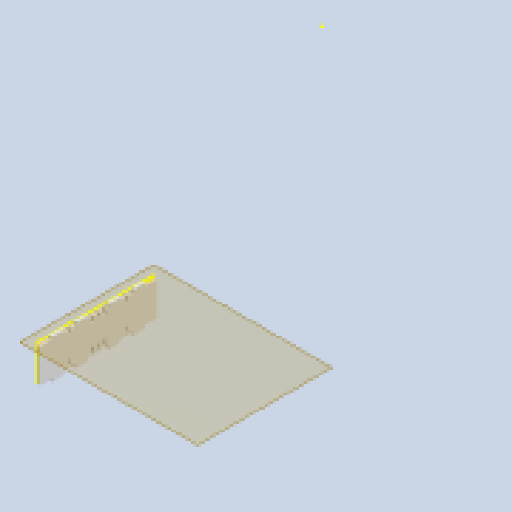
# Autodesk Inventor part: стенка
Saved by Autodesk Inventor 2024.2 (Build 282272000, 272)
## iProperties
Created: 2025-12-09
Part Number: стенка
Material: Типовые
Document SubType Name: Modeling
Designer: katya_notebook
Mass: 65.1748 g
Surface Area: 247.334 cm^2
Volume: 65.1748 cm^3
Density: 1 g/cm^3
Appearance: По умолчанию
Author: katya_notebook
Autodesk Inventor part; units mm, degrees
ref_plane "YZ Plane" through (0, 0, 0) normal (1, 0, 0) x (0, 1, 0)
ref_plane "XZ Plane" through (0, 0, 0) normal (0, 1, 0) x (-1, 0, 0)
ref_plane "XY Plane" through (0, 0, 0) normal (0, 0, 1) x (1, 0, 0)
ref_plane "РабПлоскость1" through (-475.2675, -216.9886, 379.0883) normal (0, 1, 0) x (-1, 0, 0)
sketch "Эскиз1" plane through (-475.2675, -216.9886, 379.0883) normal (0, 1, 0) x (-1, 0, 0)
  line L0 (135, 97.5) -> (129, 97.5)
  line L1 (129, 97.5) -> (129, -97.5)
  line L2 (129, -97.5) -> (135, -97.5)
  line L3 (135, -97.5) -> (135, 97.5)
  line L4 (135, -97.5) -> (135, 97.5) projected
  line L5 (135, 97.5) -> (62.5237, 97.5) projected
  line L6 (62.5237, -97.5) -> (135, -97.5) projected
  point P0 (-475.2675, -379.0883)
  dimension "d0" = 0
  dimension "d1" = 6
  dimension "d2" = 0
  dimension "d3" = 0
  constraints: 8 end point, 2 parallel, 1 horizontal, 1 perpendicular
  measures "d0" distance between parallel lines of L4 L3
  measures "d1" distance of L0.start L0.end
  measures "d2" distance between parallel lines of L6 L2
  measures "d3" distance between parallel lines of L0 L5
ref_plane "РабПлоскость2" through (-610.2675, -276.6936, 277.5883) normal (0, 1, 0) x (0, 0, 1)
extrude "Выдавливание1" add sketch "Эскиз1" against normal up to surface (59.705 mm away)
sketch "Эскиз2" plane through (-610.2675, -216.9886, 281.5883) normal (-1, 0, 0) x (0, 0, 1)
  line L0 (0, -4) -> (20, -4) projected
  line L1 (195, 0) -> (195, -59.705) projected
  line L2 (0, 0) -> (195, 0) projected
  line L3 (0, 0) -> (0, -59.705) projected
  point P0 (-281.5883, 216.9886)
  point P1 (195, -59.705)
  constraints: 1 other
sketch "Эскиз3" plane through (-610.2675, -276.6936, 281.5883) normal (-1, 0, 0) x (0, 0, 1)
  line L0 (195, 0) -> (0, 0) projected
  line L1 (175, 0) -> (155, 0)
  line L2 (155, 0) -> (155, -5)
  line L3 (155, -5) -> (175, -5)
  line L4 (175, -5) -> (175, 0)
  line L5 (195, 59.705) -> (195, 0) projected
  line L6 (135, 0) -> (115, 0)
  line L7 (115, 0) -> (115, -5)
  line L8 (115, -5) -> (135, -5)
  line L9 (135, -5) -> (135, 0)
  line L10 (20, 0) -> (40, 0)
  line L11 (40, 0) -> (40, -5)
  line L12 (40, -5) -> (20, -5)
  line L13 (20, -5) -> (20, 0)
  line L14 (60, 0) -> (80, 0)
  line L15 (80, 0) -> (80, -5)
  line L16 (80, -5) -> (60, -5)
  line L17 (60, -5) -> (60, 0)
  line L18 (97.5, 27.8525) -> (226.4185, 27.8525)
  line L19 (195, 55.705) -> (0, 55.705)
  line L20 (175, 55.705) -> (155, 55.705)
  line L21 (155, 55.705) -> (155, 60.705)
  line L22 (155, 60.705) -> (175, 60.705)
  line L23 (175, 60.705) -> (175, 55.705)
  line L24 (135, 55.705) -> (115, 55.705)
  line L25 (115, 55.705) -> (115, 60.705)
  line L26 (115, 60.705) -> (135, 60.705)
  line L27 (135, 60.705) -> (135, 55.705)
  line L28 (20, 55.705) -> (40, 55.705)
  line L29 (40, 55.705) -> (40, 60.705)
  line L30 (40, 60.705) -> (20, 60.705)
  line L31 (20, 60.705) -> (20, 55.705)
  line L32 (60, 55.705) -> (80, 55.705)
  line L33 (80, 55.705) -> (80, 60.705)
  line L34 (80, 60.705) -> (60, 60.705)
  line L35 (60, 60.705) -> (60, 55.705)
  point P0 (-281.5883, 276.6936)
  point P1 (40, 55.705)
  point P2 (80, 55.705)
  point P3 (40, 0)
  point P4 (80, 0)
  point P5 (115, 55.705)
  point P6 (155, 55.705)
  point P7 (115, 0)
  point P8 (155, 0)
  dimension "d8" = 5
  dimension "d9" = 20
  dimension "d10" = 20
  dimension "d11" = 20
  dimension "d12" = 20
  dimension "d13" = 5
  dimension "d14" = 20
  dimension "d15" = 20
  dimension "d16" = 20
  dimension "d17" = 20
  dimension "d43" = 5
  constraints: 68 end point, 17 symmetric about line, 8 parallel, 8 point on line, 5 horizontal, 4 perpendicular
  measures "d8" distance of L3.end L1.start
  measures "d9" distance of L2.end L3.end
  measures "d10" distance of L0.start L1.start
  measures "d11" distance of L7.end L8.end
  measures "d12" distance of L1.end L6.start
  measures "d13" distance of L10.end L11.end
  measures "d14" distance of L11.end L12.end
  measures "d15" distance of L10.start L0.end
  measures "d16" distance of L15.end L16.end
  measures "d17" distance of L14.start L10.end
  measures "d43" distance of L16.end L14.start
extrude "Выдавливание3" add sketch "Эскиз3" against normal blind 6
sketch "Эскиз4" plane through (-610.2675, -276.6936, 281.5883) normal (-1, 0, 0) x (0, 0, 1)
  point P0 (-281.5883, 276.6936)
sketch "Эскиз5" plane through (-610.2675, -276.6936, 281.5883) normal (-1, 0, 0) x (0, 0, 1)
  point P0 (-281.5883, 276.6936)
sketch "Эскиз6" plane through (-610.2675, -276.6936, 281.5883) normal (-1, 0, 0) x (0, 0, 1)
  line L0 (111.125, 1.5) -> (104.625, 1.5)
  line L1 (104.625, 1.5) -> (104.625, 4.5)
  line L2 (104.625, 4.5) -> (111.125, 4.5)
  line L3 (111.125, 4.5) -> (111.125, 1.5)
  line L4 (115, 0) -> (115, -5) projected
  line L5 (100.75, 1.5) -> (94.25, 1.5)
  line L6 (94.25, 1.5) -> (94.25, 4.5)
  line L7 (94.25, 4.5) -> (100.75, 4.5)
  line L8 (100.75, 4.5) -> (100.75, 1.5)
  line L9 (90.375, 1.5) -> (83.875, 1.5)
  line L10 (83.875, 1.5) -> (83.875, 4.5)
  line L11 (83.875, 4.5) -> (90.375, 4.5)
  line L12 (90.375, 4.5) -> (90.375, 1.5)
  line L13 (111.125, 3) -> (104.625, 3)
  line L14 (115, 0) -> (80, 0) projected
  line L15 (106.125, 6) -> (109.625, 6)
  line L16 (109.625, 6) -> (109.625, 0)
  line L17 (109.625, 0) -> (106.125, 0)
  line L18 (106.125, 0) -> (106.125, 6)
  line L19 (106.125, 6) -> (109.625, 0) construction
  line L20 (109.625, 6) -> (106.125, 0) construction
  line L21 (100.75, 3) -> (94.25, 3)
  line L22 (97.5, 1.5) -> (97.5, 4.5)
  line L23 (90.375, 3) -> (83.875, 3)
  line L24 (87.125, 1.5) -> (87.125, 4.5)
  line L25 (95.75, 6) -> (99.25, 6)
  line L26 (99.25, 6) -> (99.25, 0)
  line L27 (99.25, 0) -> (95.75, 0)
  line L28 (95.75, 0) -> (95.75, 6)
  line L29 (95.75, 6) -> (99.25, 0) construction
  line L30 (99.25, 6) -> (95.75, 0) construction
  line L31 (85.375, 6) -> (88.875, 6)
  line L32 (88.875, 6) -> (88.875, 0)
  line L33 (88.875, 0) -> (85.375, 0)
  line L34 (85.375, 0) -> (85.375, 6)
  line L35 (85.375, 6) -> (88.875, 0) construction
  line L36 (88.875, 6) -> (85.375, 0) construction
  line L37 (148.25, 1.5) -> (141.75, 1.5)
  line L38 (141.75, 1.5) -> (141.75, 4.5)
  line L39 (141.75, 4.5) -> (148.25, 4.5)
  line L40 (148.25, 4.5) -> (148.25, 1.5)
  line L41 (148.25, 3) -> (141.75, 3)
  line L42 (143.25, 12) -> (146.75, 12)
  line L43 (146.75, 12) -> (146.75, -6)
  line L44 (146.75, -6) -> (143.25, -6)
  line L45 (143.25, -6) -> (143.25, 12)
  line L46 (143.25, 12) -> (146.75, -6) construction
  line L47 (146.75, 12) -> (143.25, -6) construction
  line L48 (155, 0) -> (155, -5) projected
  line L49 (53.25, 1.5) -> (46.75, 1.5)
  line L50 (46.75, 1.5) -> (46.75, 4.5)
  line L51 (46.75, 4.5) -> (53.25, 4.5)
  line L52 (53.25, 4.5) -> (53.25, 1.5)
  line L53 (53.25, 3) -> (46.75, 3)
  line L54 (48.25, 12) -> (51.75, 12)
  line L55 (51.75, 12) -> (51.75, -6)
  line L56 (51.75, -6) -> (48.25, -6)
  line L57 (48.25, -6) -> (48.25, 12)
  line L58 (48.25, 12) -> (51.75, -6) construction
  line L59 (51.75, 12) -> (48.25, -6) construction
  line L60 (60, 0) -> (60, -5) projected
  line L61 (195, 59.705) -> (195, 0) projected
  line L62 (195, 29.8525) -> (88.875, 29.8525)
  line L63 (111.125, 58.205) -> (104.625, 58.205)
  line L64 (104.625, 58.205) -> (104.625, 55.205)
  line L65 (104.625, 55.205) -> (111.125, 55.205)
  line L66 (111.125, 55.205) -> (111.125, 58.205)
  line L67 (115, 59.705) -> (115, 64.705)
  line L68 (100.75, 58.205) -> (94.25, 58.205)
  line L69 (94.25, 58.205) -> (94.25, 55.205)
  line L70 (94.25, 55.205) -> (100.75, 55.205)
  line L71 (100.75, 55.205) -> (100.75, 58.205)
  line L72 (90.375, 58.205) -> (83.875, 58.205)
  line L73 (83.875, 58.205) -> (83.875, 55.205)
  line L74 (83.875, 55.205) -> (90.375, 55.205)
  line L75 (90.375, 55.205) -> (90.375, 58.205)
  line L76 (111.125, 56.705) -> (104.625, 56.705)
  line L77 (115, 59.705) -> (80, 59.705)
  line L78 (106.125, 53.705) -> (109.625, 53.705)
  line L79 (109.625, 53.705) -> (109.625, 59.705)
  line L80 (109.625, 59.705) -> (106.125, 59.705)
  line L81 (106.125, 59.705) -> (106.125, 53.705)
  line L82 (106.125, 53.705) -> (109.625, 59.705) construction
  line L83 (109.625, 53.705) -> (106.125, 59.705) construction
  line L84 (100.75, 56.705) -> (94.25, 56.705)
  line L85 (97.5, 58.205) -> (97.5, 55.205)
  line L86 (90.375, 56.705) -> (83.875, 56.705)
  line L87 (87.125, 58.205) -> (87.125, 55.205)
  line L88 (95.75, 53.705) -> (99.25, 53.705)
  line L89 (99.25, 53.705) -> (99.25, 59.705)
  line L90 (99.25, 59.705) -> (95.75, 59.705)
  line L91 (95.75, 59.705) -> (95.75, 53.705)
  line L92 (95.75, 53.705) -> (99.25, 59.705) construction
  line L93 (99.25, 53.705) -> (95.75, 59.705) construction
  line L94 (85.375, 53.705) -> (88.875, 53.705)
  line L95 (88.875, 53.705) -> (88.875, 59.705)
  line L96 (88.875, 59.705) -> (85.375, 59.705)
  line L97 (85.375, 59.705) -> (85.375, 53.705)
  line L98 (85.375, 53.705) -> (88.875, 59.705) construction
  line L99 (88.875, 53.705) -> (85.375, 59.705) construction
  line L100 (146.75, 65.705) -> (143.25, 65.705)
  line L101 (146.75, 47.705) -> (146.75, 65.705)
  line L102 (146.75, 47.705) -> (143.25, 65.705) construction
  line L103 (143.25, 47.705) -> (146.75, 65.705) construction
  line L104 (143.25, 65.705) -> (143.25, 47.705)
  line L105 (141.75, 58.205) -> (141.75, 55.205)
  line L106 (148.25, 58.205) -> (141.75, 58.205)
  line L107 (148.25, 55.205) -> (148.25, 58.205)
  line L108 (141.75, 55.205) -> (148.25, 55.205)
  line L109 (148.25, 56.705) -> (141.75, 56.705)
  line L110 (143.25, 47.705) -> (146.75, 47.705)
  line L111 (155, 59.705) -> (155, 64.705)
  line L112 (51.75, 65.705) -> (48.25, 65.705)
  line L113 (51.75, 47.705) -> (51.75, 65.705)
  line L114 (51.75, 47.705) -> (48.25, 65.705) construction
  line L115 (48.25, 47.705) -> (51.75, 65.705) construction
  line L116 (48.25, 65.705) -> (48.25, 47.705)
  line L117 (46.75, 58.205) -> (46.75, 55.205)
  line L118 (53.25, 58.205) -> (46.75, 58.205)
  line L119 (53.25, 55.205) -> (53.25, 58.205)
  line L120 (46.75, 55.205) -> (53.25, 55.205)
  line L121 (53.25, 56.705) -> (46.75, 56.705)
  line L122 (48.25, 47.705) -> (51.75, 47.705)
  line L123 (60, 59.705) -> (60, 64.705)
  line L124 (109.625, 6) -> (106.125, 6)
  line L125 (106.125, 6) -> (106.125, 12)
  line L126 (106.125, 12) -> (109.625, 12)
  line L127 (109.625, 12) -> (109.625, 6)
  line L128 (99.25, 6) -> (95.75, 6)
  line L129 (95.75, 6) -> (95.75, 12)
  line L130 (95.75, 12) -> (99.25, 12)
  line L131 (99.25, 12) -> (99.25, 6)
  line L132 (88.875, 6) -> (85.375, 6)
  line L133 (85.375, 6) -> (85.375, 12)
  line L134 (85.375, 12) -> (88.875, 12)
  line L135 (88.875, 12) -> (88.875, 6)
  line L136 (109.625, 53.705) -> (106.125, 53.705)
  line L137 (106.125, 53.705) -> (106.125, 47.705)
  line L138 (106.125, 47.705) -> (109.625, 47.705)
  line L139 (109.625, 47.705) -> (109.625, 53.705)
  line L140 (99.25, 53.705) -> (95.75, 53.705)
  line L141 (95.75, 53.705) -> (95.75, 47.705)
  line L142 (95.75, 47.705) -> (99.25, 47.705)
  line L143 (99.25, 47.705) -> (99.25, 53.705)
  line L144 (88.875, 53.705) -> (85.375, 53.705)
  line L145 (85.375, 53.705) -> (85.375, 47.705)
  line L146 (85.375, 47.705) -> (88.875, 47.705)
  line L147 (88.875, 47.705) -> (88.875, 53.705)
  point P0 (-281.5883, 276.6936)
  point P1 (115, -2.5)
  point P2 (107.875, 11.6549)
  point P3 (107.875, 3)
  point P4 (97.5, 3)
  point P5 (87.125, 3)
  point P6 (149.0518, 14.6563)
  point P7 (145, 3)
  point P8 (155, -2.5)
  point P9 (49.2049, 25.9501)
  point P10 (50, 3)
  point P11 (60, -2.5)
  point P12 (48.25, 4.5)
  point P13 (48.25, 1.5)
  point P14 (51.75, 1.5)
  point P15 (51.75, 4.5)
  point P16 (88.875, 4.5)
  point P17 (85.375, 4.5)
  point P18 (85.375, 1.5)
  point P19 (85.375, 0)
  point P20 (88.875, 1.5)
  point P21 (95.75, 1.5)
  point P22 (95.75, 0)
  point P23 (99.25, 1.5)
  point P24 (99.25, 4.5)
  point P25 (95.75, 4.5)
  point P26 (106.125, 1.5)
  point P27 (106.125, 0)
  point P28 (109.625, 1.5)
  point P29 (109.625, 4.5)
  point P30 (106.125, 4.5)
  point P31 (143.25, 1.5)
  point P32 (146.75, 1.5)
  point P33 (146.75, 4.5)
  point P34 (143.25, 4.5)
  point P35 (195, 55.705)
  point P36 (115, 62.205)
  point P37 (107.875, 48.0501)
  point P38 (107.875, 56.705)
  point P39 (97.5, 56.705)
  point P40 (87.125, 56.705)
  point P41 (145, 56.705)
  point P42 (149.0518, 45.0486)
  point P43 (155, 62.205)
  point P44 (50, 56.705)
  point P45 (60, 62.205)
  point P46 (51.75, 55.205)
  point P47 (51.75, 58.205)
  point P48 (48.25, 58.205)
  point P49 (48.25, 55.205)
  point P50 (88.875, 55.205)
  point P51 (88.875, 58.205)
  point P52 (85.375, 55.705)
  point P53 (85.375, 58.205)
  point P54 (85.375, 55.205)
  point P55 (99.25, 55.205)
  point P56 (99.25, 58.205)
  point P57 (95.75, 58.205)
  point P58 (95.75, 55.205)
  point P59 (106.125, 58.205)
  point P60 (106.125, 55.205)
  point P61 (109.625, 55.205)
  point P62 (109.625, 58.205)
  point P63 (143.25, 58.205)
  point P64 (143.25, 55.205)
  point P65 (146.75, 55.205)
  point P66 (146.75, 58.205)
  point P67 (85.375, 59.705)
  point P68 (85.375, 53.705)
  point P69 (95.75, 53.705)
  point P70 (106.125, 53.705)
  point P71 (85.375, 6)
  point P72 (95.75, 6)
  point P73 (106.125, 6)
  dimension "d1" = 6
  dimension "d20" = 6.5
  dimension "d21" = 3
  dimension "d22" = 3.875
  dimension "d23" = 6.5
  dimension "d24" = 3
  dimension "d25" = 3.875
  dimension "d26" = 6.5
  dimension "d27" = 3
  dimension "d28" = 3.875
  dimension "d29" = 3
  dimension "d30" = 3.5
  dimension "d31" = 3.5
  dimension "d32" = 3.5
  dimension "d33" = 6.5
  dimension "d34" = 3
  dimension "d35" = 3.5
  dimension "d36" = 8.25
  dimension "d37" = 6.5
  dimension "d38" = 3
  dimension "d39" = 3.5
  dimension "d40" = 8.25
  dimension "d46" = 6
  dimension "d47" = 6
  constraints: 286 end point, 71 symmetric about line, 33 midpoint, 32 parallel, 18 perpendicular, 17 horizontal, 8 collinear, 8 point on line
  measures "d20" distance of L0.start L0.end
  measures "d21" distance of L0.end L1.end
  measures "d22" horizontal distance of L13.start point (115, -2.5)
  measures "d23" distance of L5.start L5.end
  measures "d24" distance of L5.end L6.end
  measures "d25" distance of L7.end L1.end
  measures "d26" distance of L9.start L9.end
  measures "d27" distance of L9.end L10.end
  measures "d28" distance of L6.end L11.end
  measures "d29" distance from line of L14 point (107.875, 3)
  measures "d30" distance of L16.end L17.end
  measures "d31" distance of L27.end L26.end
  measures "d32" distance of L33.end L32.end
  measures "d33" distance of L37.start L38.start
  measures "d34" distance of L38.start L38.end
  measures "d35" distance of L44.start L44.end
  measures "d36" distance from line of L43 point (155, -2.5)
  measures "d37" distance of L49.start L50.start
  measures "d38" distance of L50.start L50.end
  measures "d39" distance of L56.start L56.end
  measures "d40" distance from line of L55 point (60, -2.5)
  measures "d46" distance of L124.end L125.end
  measures "d47" distance of L136.end L137.end
extrude "Выдавливание4" cut sketch "Эскиз6" against normal blind 6
sketch "Эскиз7" plane through (-610.2675, -276.6936, 281.5883) normal (-1, 0, 0) x (0, 0, 1)
  line L0 (175, 55.705) -> (195, 55.705) projected
  line L1 (195, 59.705) -> (195, 0) projected
  line L2 (175, 59.705) -> (195, 59.705) projected
  line L3 (175, 59.705) -> (175, 55.705) projected
  line L4 (155, 55.705) -> (155, 59.705) projected
  line L5 (135, 55.705) -> (155, 55.705) projected
  line L6 (135, 59.705) -> (135, 55.705) projected
  line L7 (135, 59.705) -> (155, 59.705) projected
  line L8 (80, 55.705) -> (115, 55.705) projected
  line L9 (115, 55.705) -> (115, 59.705) projected
  line L10 (80, 59.705) -> (80, 55.705) projected
  line L11 (80, 59.705) -> (115, 59.705) projected
  line L12 (60, 55.705) -> (60, 59.705) projected
  line L13 (40, 55.705) -> (60, 55.705) projected
  line L14 (40, 59.705) -> (60, 59.705) projected
  line L15 (40, 59.705) -> (40, 55.705) projected
  line L16 (0, 55.705) -> (20, 55.705) projected
  line L17 (20, 55.705) -> (20, 59.705) projected
  line L18 (0, 59.705) -> (20, 59.705) projected
  line L19 (0, 59.705) -> (0, 0) projected
  point P0 (-281.5883, 276.6936)
  point P1 (175, 59.705)
extrude "Выдавливание5" cut sketch "Эскиз7" against normal blind 6
